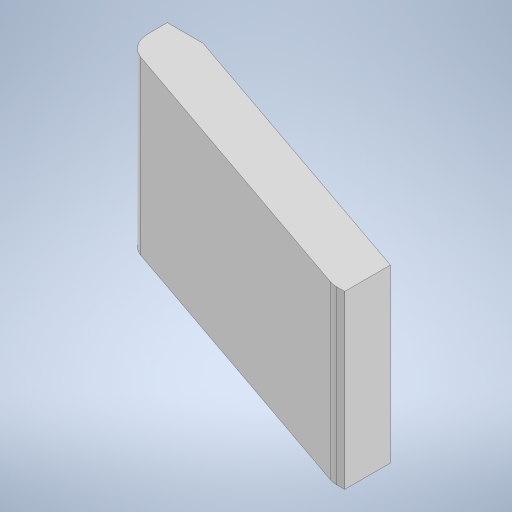
# Autodesk Inventor part: Part4 x 2
Saved by Autodesk Inventor 2023.1 (Build 271208000, 208)
## iProperties
Created: 2022-10-25
Part Number: Part4 x 2
Material: Generic
Document SubType Name: Modeling
Designer: jshin23
Density: 1 g/cm^3
Appearance: Default
Author: jshin23
Autodesk Inventor part; units mm, degrees
ref_plane "YZ Plane" through (0, 0, 0) normal (1, 0, 0) x (0, 1, 0)
ref_plane "XZ Plane" through (0, 0, 0) normal (0, 1, 0) x (-1, 0, 0)
ref_plane "XY Plane" through (0, 0, 0) normal (0, 0, 1) x (1, 0, 0)
sketch "Sketch1" plane through (0, 0, 0) normal (0, 1, 0) x (-1, 0, 0)
  line L0 (110.0582, -50.5961) -> (122.7582, -50.5961)
  line L1 (122.7582, -37.2525) -> (122.7582, -50.5961)
  line L2 (122.7582, -37.2525) -> (12.7, 0.6436)
  line L3 (12.7, 0.6436) -> (8.4582, 0.6436)
  line L4 (8.4582, 0.6436) -> (8.4582, -15.6124)
  line L5 (8.4582, -15.6124) -> (110.0582, -50.5961)
  point P0 (122.7582, -43.9243)
  dimension "d17" = 4.2418
  dimension "d18" = 114.3
  dimension "d19" = 109
  dimension "d21" = 12.7
  dimension "d22" = 16.256
  constraints: 12 end point, 2 horizontal, 1 midpoint, 1 parallel, 1 perpendicular, 1 vertical
  measures "d17" distance of L2.end L3.end
  measures "d18" distance between parallel lines of L4 L1
  measures "d19" angle of L1 L2
  measures "d21" distance of L0.start L0.end
  measures "d22" distance of L3.end L4.end
extrude "Extrusion1" add sketch "Sketch1" along normal blind 60.96
fillet "Fillet2" radius 8.89 2 edges at (-12.7, 30.48, 0.6436) (-122.7582, 30.48, -37.2525)
body "Solid1"
